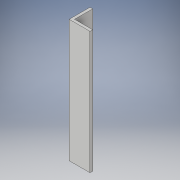
# Autodesk Inventor part: FrameThickBracket
Saved by Autodesk Inventor 2019 (Build 230136000, 136)
## iProperties
Created: 2018-08-17
Part Number: FrameThickBracket
Material: Generic
Document SubType Name: Modeling
Designer: Kitte_X
Density: 1 g/cm^3
Appearance: Default
Author: Kitte_X
Autodesk Inventor part; units mm, degrees
ref_plane "YZ Plane" through (0, 0, 0) normal (1, 0, 0) x (0, 1, 0)
ref_plane "XZ Plane" through (0, 0, 0) normal (0, 1, 0) x (-1, 0, 0)
ref_plane "XY Plane" through (0, 0, 0) normal (0, 0, 1) x (1, 0, 0)
sketch "Sketch1" plane through (0, 0, 0) normal (0, 1, 0) x (-1, 0, 0)
  line L0 (24.6842, 32.5) -> (-25.3158, 32.5)
  line L1 (-25.3158, 32.5) -> (-25.3158, 26)
  line L2 (-25.3158, 26) -> (18.1842, 26)
  line L3 (18.1842, 26) -> (18.1842, -17.5)
  line L4 (18.1842, -17.5) -> (24.6842, -17.5)
  line L5 (24.6842, -17.5) -> (24.6842, 32.5)
  point P0 (0, 0)
  dimension "d0" = 6.5
  dimension "d1" = 6.5
  dimension "d2" = 50
  dimension "d3" = 50
  constraints: 13 end point, 5 perpendicular, 1 horizontal
  measures "d0" distance between parallel lines of L2 L0
  measures "d1" distance between parallel lines of L5 L3
  measures "d2" distance of L4.end L0.start
  measures "d3" distance of L0.start L0.end
extrude "Extrusion1" add sketch "Sketch1" along normal blind 294
body "Solid1"
